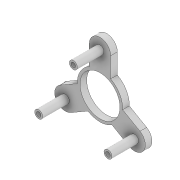
# Autodesk Inventor part: Planetery gearbox port
Saved by Autodesk Inventor 2020.3 (Build 243373010, 373A)
## iProperties
Created: 2021-05-04
Part Number: Planetery gearbox port
Material: Generic
Document SubType Name: Modeling
Designer: marti
Density: 1 g/cm^3
Appearance: Default
Author: marti
Autodesk Inventor part; units mm, degrees
ref_plane "YZ Plane" through (0, 0, 0) normal (1, 0, 0) x (0, 1, 0)
ref_plane "XZ Plane" through (0, 0, 0) normal (0, 1, 0) x (-1, 0, 0)
ref_plane "XY Plane" through (0, 0, 0) normal (0, 0, 1) x (1, 0, 0)
sketch "Sketch3" plane through (0, 0, 0) normal (0, 0, 1) x (1, 0, 0)
  circle A0 centre (0, 0) radius 7.5
  circle A1 centre (0, 15) radius 4
  line L0 (0, 0) -> (0, 15)
  line L1 (-4, 15) -> (-4, 6.3443)
  line L2 (4, 15) -> (4, 6.3443)
  circle A2 centre (0, 0) radius 8.5
  circle A3 centre (-12.9904, -7.5) radius 4
  line L3 (-14.9904, -4.0359) -> (-7.4943, 0.292)
  line L4 (-10.9904, -10.9641) -> (-3.4943, -6.6362)
  circle A4 centre (12.9904, -7.5) radius 4
  line L5 (10.9904, -10.9641) -> (3.4943, -6.6362)
  line L6 (14.9904, -4.0359) -> (7.4943, 0.292)
  point P0 (-4, 7.5)
  point P1 (4, 7.5)
  point P2 (8.4952, -0.2859)
  point P3 (4.4952, -7.2141)
  point P4 (-4.4952, -7.2141)
  point P5 (-8.4952, -0.2859)
  dimension "d13" = 15
  dimension "d14" = 8
  dimension "d17" = 15
  dimension "d26" = 17
  dimension "d29" = 360
  constraints: 14 end point, 8 point on circle, 5 centre point, 3 coincident, 3 vertical, 2 tangent, 25 other
  measures "d13" diameter of A0
  measures "d14" diameter of A1
  measures "d17" distance of L0.start L0.end
  measures "d26" diameter of A2
extrude "Extrusion3" add sketch "Sketch3" against normal blind 2.5 contours A0 L6 A2 L5 | A0 L2 A2 L6 | L5 A2 L4 A0 | A0 L0 A2 L2 | L6 A4 L5 A2 | L4 A2 L3 A0 | A0 L1 A2 L0 | A2 L0 A1 L2 | A4 | L3 A2 L1 A0 | L4 A3 L3 A2 | A2 L1 A1 L0 | A1 | A3
sketch "Sketch4" plane through (0, 0, 0) normal (0, 0, 1) x (1, 0, 0)
  arc A0 (4, 15) -> (-4, 15) centre (0, 15) ccw projected
  circle A1 centre (0, 15) radius 1.5
  point P0 (0, 0)
  dimension "d20" = 3
  constraints: 1 centre point, 1 coincident
  measures "d20" diameter of A1
extrude "Extrusion4" add sketch "Sketch4" along normal blind 10
sketch "Sketch5" plane through (0, 0, 0) normal (0, 0, 1) x (1, 0, 0)
  circle A0 centre (0, 0) radius 7.5
  dimension "d23" = 15
  constraints: 1 centre point, 1 coincident
  measures "d23" diameter of A0
pattern_circular "Circular Pattern1" count 3 over 360 about axis through (0, 0, -10) along (0, 0, 1) of "Extrusion4"
sketch "Sketch6" plane through (0, 15, 10) normal (0, 0, 1) x (1, 0, 0)
  circle A0 centre (0, 0) radius 1.5 projected
  circle A1 centre (-12.9904, -22.5) radius 1.5 projected
  circle A2 centre (12.9904, -22.5) radius 1.5 projected
  point P0 (0, -15)
  constraints: 3 coincident
hole "Hole1" at (0, 15, 10) at (-12.9904, -7.5, 10) at (12.9904, -7.5, 10) direction (0, 0, -1) diameter 1.7294 depth 10 tip angle 118 thread size "M2x0.25" class "6H" standard "ISO Metric profile"
body "Solid2"
